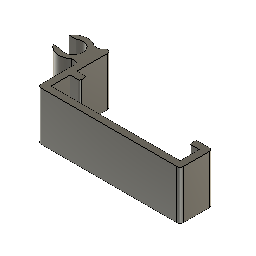
Laser air tube clip v11 (Autodesk Fusion 360 design; units mm, degrees)
Autodesk Fusion 360 part; units mm, degrees
sketch "Sketch1" plane through (0, 0, 0) normal (0, 0, 1) x (1, 0, 0)
  line L0 (0, 0) -> (40, 0)
  line L1 (40, 0) -> (40, 6)
  line L2 (0, 6) -> (0, 0)
  line L3 (37, 7.5) -> (37, 6.5)
  line L4 (3, 6.5) -> (3, 7.5)
  line L5 (42, 7) -> (42, -1)
  line L6 (41, -2) -> (-1, -2)
  line L7 (-2, -1) -> (-2, 8)
  line L8 (0, 8) -> (3, 8)
  line L9 (37, 8) -> (41, 8)
  line L10 (0, 8) -> (3, 8)
  line L11 (37, 8) -> (40, 8)
  line L12 (40, 8) -> (37.5, 8)
  line L13 (2.5, 8) -> (0, 8)
  line L14 (40, 6) -> (37.5, 6)
  line L15 (2.5, 6) -> (0, 6)
  arc A0 (3, 7.5) -> (2.5, 8) centre (2.5, 7.5) ccw
  arc A1 (2.5, 6) -> (3, 6.5) centre (2.5, 6.5) ccw
  arc A2 (37.5, 8) -> (37, 7.5) centre (37.5, 7.5) ccw
  arc A3 (37, 6.5) -> (37.5, 6) centre (37.5, 6.5) ccw
  arc A4 (-2, -1) -> (-1, -2) centre (-1, -1) ccw
  arc A5 (41, -2) -> (42, -1) centre (41, -1) ccw
  arc A6 (42, 7) -> (41, 8) centre (41, 7) ccw
  line L16 (0, 8) -> (0, 17.5)
  line L17 (-1, 18.5) -> (-1, 18.5)
  line L18 (-2, 9.5781) -> (-2, 8)
  line L19 (-3, 10.5781) -> (-4.0783, 10.5781)
  line L20 (-4.0783, 17.4226) -> (-2.7745, 17.4226)
  line L21 (-8.6583, 11.5) -> (-10.7417, 11.5)
  line L22 (-10.7417, 16.5) -> (-8.6583, 16.5)
  line L23 (-8, 11.5) -> (-14, 16.5) construction
  line L24 (-14, 11.5) -> (-8, 16.5) construction
  arc A7 (-8.6583, 11.5) -> (-8.6583, 16.5) centre (-7, 14) ccw
  arc A8 (-11.482, 14.4017) -> (-11.482, 13.5983) centre (-7, 14) ccw
  arc A9 (-10.7417, 11.5) -> (-10.7417, 16.5) centre (-7, 14) ccw
  arc A10 (-2, 9.5781) -> (-3, 10.5781) centre (-3, 9.5781) ccw
  line L25 (-2, 17.5) -> (-2, 17.4226)
  arc A11 (-1, 18.5) -> (-1.8873, 17.9613) centre (-1, 17.5) ccw
  arc A12 (0, 17.5) -> (-1, 18.5) centre (-1, 17.5) ccw
  arc A13 (-2.7745, 17.4226) -> (-1.8873, 17.9613) centre (-2.7745, 18.4226) ccw
  point P0 (42, 8)
  point P1 (-2, -2)
  point P2 (-2, 18.5)
  point P3 (-11, 14)
  dimension "d1" = 40
  dimension "d2" = 8
  dimension "d3" = 40
  dimension "d4" = 2
  dimension "d7" = 44
  dimension "d8" = 10
  dimension "d9" = 2
  dimension "d10" = 2
  dimension "d11" = 0.5
  dimension "d12" = 0.5
  dimension "d13" = 1
  dimension "d25" = 1
  dimension "d26" = 2
  dimension "d27" = 10.5
  dimension "d28" = 6
  dimension "d29" = 9
  dimension "d30" = 6
  dimension "d31" = 5
  dimension "d32" = 1
  dimension "d33" = 1
  dimension "d34" = 1
  dimension "d35" = 1
  constraint horizontal L0
  constraint vertical L1
  constraint horizontal L12
  constraint vertical L2
  constraint coincident L0.start L2.end
  constraint horizontal L10
  constraint horizontal L14
  constraint vertical L3
  constraint vertical L4
  constraint coincident L8.end L12
  constraint horizontal L8
  constraint vertical L5
  constraint horizontal L6
  constraint vertical L7
  constraint collinear L8 L9
  constraint collinear L10 L11
  constraint collinear L12 L13
  constraint collinear L14 L15
  constraint coincident L8.end L4
  constraint tangent L13 A0
  constraint tangent L4 A0
  constraint tangent L15 A1
  constraint tangent L4 A1
  constraint equal A0 A1
  constraint coincident L9.start L3
  constraint tangent L12 A2
  constraint tangent L3 A2
  constraint tangent L14 A3
  constraint tangent L3 A3
  constraint equal A2 A3
  constraint coincident P1 L6
  constraint coincident P1 L7
  constraint tangent L6 A4
  constraint tangent L7 A4
  constraint tangent L5 A5
  constraint tangent L6 A5
  constraint equal A4 A5
  constraint coincident P0 L5
  constraint coincident P0 L9
  constraint tangent L5 A6
  constraint tangent L9 A6
  constraint vertical L16
  constraint vertical L18
  constraint concentric A7 A8
  constraint horizontal L19
  constraint horizontal L20
  constraint coincident L20.start A8
  constraint horizontal L21
  constraint parallel L21 L22
  constraint coincident L23 P3
  constraint coincident L24 P3
  constraint coincident L23 A8.start
  constraint coincident L24 A8.end
  constraint concentric A8 A9
  constraint coincident P2 L18
  constraint tangent L18 A10
  constraint tangent L19 A10
  constraint coincident P2 L25
  constraint tangent L25 A11
  constraint tangent L16 A12
  constraint tangent A11 A13
  constraint tangent L20 A13
  measures "d1" distance of L0.start L0.end
  measures "d2" distance of L0.start L8.start
  measures "d3" distance of L8.start L11.end
  measures "d4" distance of L8.start L2.start
  measures "d7" distance of L7.end P0
  measures "d8" distance of L7.end P1
  measures "d9" distance of L2 L7
  measures "d10" distance of L0 L6
  measures "d11" radius of A0
  measures "d12" radius of A2
  measures "d13" radius of A4
  measures "d25" radius of A6
  measures "d26" distance of L7.end L8.start
  measures "d27" distance of L7.end P2
  measures "d28" diameter of A7
  measures "d29" diameter of A8
  measures "d30" distance of L23.end L24.end
  measures "d31" distance of L24.start L23.end
  measures "d32" radius of A10
  measures "d33" radius of A11
  measures "d34" radius of A12
  measures "d35" radius of A13
extrude "Extrude1" add sketch "Sketch1" along normal blind 15
